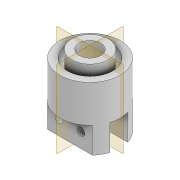
# Autodesk Inventor part: Feather_0_clip
Saved by Autodesk Inventor 2022 (Build 260153000, 153)
## iProperties
Created: 2022-07-26
Part Number: Feather_0_clip
Material: Generic
Document SubType Name: Modeling
Designer: dell
Density: 1 g/cm^3
Appearance: Default
Author: dell
Autodesk Inventor part; units mm, degrees
ref_plane "XZ Plane" through (0, 0, 0) normal (0, 1, 0) x (-1, 0, 0)
sketch "Sketch1" plane through (0, 0, 0) normal (0, 1, 0) x (-1, 0, 0)
  circle A0 centre (0, 0) radius 6.1
  circle A1 centre (0, 0) radius 4.9
  circle A2 centre (0, 0) radius 8.1
  circle A3 centre (0, 0) radius 2.9
  dimension "d0" = 12.2
  dimension "d1" = 9.8
  dimension "d2" = 2
  dimension "d5" = 2
  constraints: 4 centre point, 2 coincident
  measures "d0" diameter of A0
  measures "d1" diameter of A1
  measures "d2" radial gap between concentric circles of A0 A2
  measures "d5" radial gap between concentric circles of A1 A3
extrude "Extrusion1" add sketch "Sketch1" along normal blind 3 contours A0 | A1 | A2 | A3
extrude "Extrusion2" add sketch "Sketch1" along normal blind 10
sketch "Sketch7" plane through (0, 0, 0) normal (0, -1, 0) x (1, 0, 0)
  circle A0 centre (0, 0) radius 8.1 projected
  line L0 (7.7363, -2.4) -> (-7.7363, -2.4)
  line L1 (-7.7363, -2.4) -> (-7.7363, -5.4)
  line L2 (-7.7363, -5.4) -> (7.7363, -5.4)
  line L3 (7.7363, -5.4) -> (7.7363, -2.4)
  line L4 (7.7363, 2.4) -> (-7.7363, 2.4)
  line L5 (-7.7363, 2.4) -> (-7.7363, 5.4)
  line L6 (-7.7363, 5.4) -> (7.7363, 5.4)
  line L7 (7.7363, 5.4) -> (7.7363, 2.4)
  point P0 (6.0374, 5.4)
  point P1 (-6.0374, 5.4)
  point P2 (-6.0374, -5.4)
  point P3 (6.0374, -5.4)
  dimension "d34" = 3
  dimension "d35" = 3
  dimension "d36" = 4.8
  dimension "d37" = 2.4
  constraints: 16 end point, 4 parallel, 4 point on circle, 2 horizontal, 2 perpendicular
  measures "d34" distance of L1.end L0.end
  measures "d35" distance of L4.end L5.end
  measures "d36" distance between parallel lines of L0 L4
  measures "d37" distance from line of point (0, 0) L0
extrude "Extrusion7" add sketch "Sketch7" along normal blind 7 contours L4 A0 L6 | A0 L2 L0
sketch "Sketch8" plane through (-6.0374, 0, 5.4) normal (0, 0, 1) x (1, 0, 0)
  circle A0 centre (3.0874, -3) radius 1.05
  circle A1 centre (8.9874, -3) radius 1.05
  line L0 (12.0748, 0) -> (0, 0) projected
  point P0 (6.0374, 0)
  dimension "d40" = 2.1
  dimension "d41" = 2.1
  dimension "d42" = 3
  dimension "d43" = 3
  dimension "d44" = 5.9
  dimension "d45" = 2.95
  constraints: 2 centre point
  measures "d40" diameter of A0
  measures "d41" diameter of A1
  measures "d42" distance from line of L0 A1.centre
  measures "d43" distance from line of L0 A0.centre
  measures "d44" distance of A0.centre A1.centre
  measures "d45" horizontal distance of point (6.037, 0) A0.centre
extrude "Extrusion8" cut sketch "Sketch8" against normal blind 20
sketch "Sketch9" plane through (0, 10, 0) normal (0, 1, 0) x (1, 0, 0)
  circle A0 centre (0, 0) radius 6.1 projected
  circle A1 centre (0, 0) radius 2.9 projected
  circle A2 centre (0, 0) radius 4.9 projected
  circle A3 centre (0, 0) radius 8.1 projected
extrude "Extrusion9" add sketch "Sketch9" along normal blind 2 contours A2
equation "\"d37\" = 0.5 * d36"
equation "\"d45\" = 0.5 * d44"
body "Solid1"
